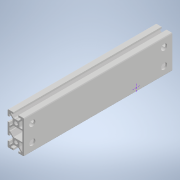
# Autodesk Inventor part: HFSF5-2040-180-LWH-RWH
Saved by Autodesk Inventor 2022 (Build 260153000, 153)
## iProperties
Category: PARTsolutions
Company: MISUMI
Created: 2022-12-05
Part Number: HFSF5-2040-180-LWH-RWH
Material: Generic
Catalog Web Link: www.cadenas.de
Description: NFS5-2040, NFSB5-2040, HFS5-2040, HFSB5-2040, CAF5-2040, NFSF5-2040, HFSF5-2040, HFSY5-2040-Aluminum Frames -5 Series-2Row Groove 20x40 mm Square -Specified Length
Vendor: MISUMI
Document SubType Name: Modeling
Designer: psAdmin
Manufacturer: MISUMI
Mass: 59.334 g
Surface Area: 583.137 cm^2
Volume: 59.334 cm^3
Density: 1 g/cm^3
Appearance: PSOLRGB-175-175-175
PSOL_IDENT_0: {$CADENAS_DATA/23d-libs/misumi/metric/38_al_extrusions_blackets/5/hfs5_2040.prj},644 {VTYP=3D},{NB=H
PSOL_IDENT_1: FSF5-2040-180-LWH-RWH},{LINA=HFSF5-2040-180-LWH-RWH},{NN=NFS5-2040, NFSB5-2040, HFS5-2040, HFSB5-204
PSOL_IDENT_2: 0, CAF5-2040, NFSF5-2040, HFSF5-2040, HFSY5-2040},{DATE=30.11.2021 06:05:55},{GEOMDATE=23.09.2021 02
PSOL_IDENT_3: :57:03},{VERSION=},{LINEID=30},{WBVAR=L,ALT1,ALT2,ALT4,ALT5,CP5,DL5,DR5,ALT6,ALT9,ALT10,ALT11,HP6,NH
PSOL_IDENT_4: L6,DL6,NHR6,DR6,ALT7,ALT8,NH9,AH,BH,CH,DH,EH,NH10,AV,BV,CV,DV,EV,NH11,AP,BP,CP,DP,EP,ALT12,ALT13,Z,N
PSOL_IDENT_5: H12,XA,XB,XC,XD,XE,NH13,YA,YB,YC,YD,YE,ALT16,HP16,DL16,DR16,ALT17,HQ17,JLP,ALT18,HQ18,KLP,ALT20},{WB
PSOL_IDENT_6: NUMERIC=L,NH9,AH,BH,CH,DH,EH,NH10,AV,BV,CV,DV,EV,NH11,AP,BP,CP,DP,EP,NH12,XA,XB,XC,XD,XE,NH13,YA,YB,
PSOL_IDENT_7: YC,YD,YE,HQ17,JLP,HQ18,KLP}  {NB=HFSF5-2040-180-LWH-RWH},{LINA=HFSF5-2040-180-LWH-RWH},{KT=DUMMY},{P
PSOL_IDENT_8: N=HFSF5-2040-180-LWH-RWH},{TPS=HFSF5-2040},{MAT=A6N01SS-T5 Aluminum Alloy},{ST=Clear Anodize},{FRMW=
PSOL_IDENT_9: 20},{FRMH=40},{FRD=4.2},{L=180},{MASS=0.93},{SA=344},{LX=1.52x10^4},{LY=5.40x10^4},{ALT1=},{M1=0},{D
PSOL_IDENT_10: PL1=0},{DPR1=0},{ALT1PN=},{ALT2=},{ALT2ALG= '','w/o End Tapping (Insert)','LHP','with LHP (Tapping o
PSOL_IDENT_11: n the Left (Insert))','RHP','with RHP (Tapping on the Right (Insert))','HPW','with HPW (Tapping on B
PSOL_IDENT_12: oth Ends (Insert))' },{M2=0},{DP2=0},{ALT2PN=},{ALT4=},{ALT4ALG= '', 'w/o SC (High Precision Cut)', '
PSOL_IDENT_13: SC', 'with SC (High Precision Cut)' },{ALT4PN=},{ALT5=},{ALT5ALG= '','w/o 45 Degree Cut','1','with 4
PSOL_IDENT_14: 5 Degree Cut' },{CP5=},{CP5ALG= '','N/A' },{DL5=},{DL5ALG= '','N/A' },{DR5=},{DR5ALG= '','N/A' },{FR
PSOL_IDENT_15: MLALT5=0},{FRMRALT5=0},{ALT5PN=},{ALT6=1},{ALT6ALG= '','w/o Fastening Location Wrench Access Hole Al
PSOL_IDENT_16: terations','1','with Fastening Location Wrench Access Hole Alterations' },{ALT9=},{ALT9ALG= '','w/o
PSOL_IDENT_17: Location Specified Wrench Access Hole Alteratons (Horizontal)','1','with Location Specified Wrench A
PSOL_IDENT_18: ccess Hole Alteratons (Horizontal)' },{ALT10=},{ALT10ALG= '','w/o Location Specified Wrench Access H
PSOL_IDENT_19: ole Alteratons (Vertical)','1','with Location Specified Wrench Access Hole Alteratons (Vertical)' },
PSOL_IDENT_20: {ALT11=},{ALT11ALG= '','w/o Location Specified Wrench Access Hole Alteratons (Crisscross)','1','with
PSOL_IDENT_21: Location Specified Wrench Access Hole Alteratons (Crisscross)' },{HP6=LR},{HP6ALG= 'L','Left','R','
PSOL_IDENT_22: Right','LR','Both Sides' },{NHL6=W},{NHL6ALG= 'C','C (Wrench Holes in Single Line)','W','W (Wrench H
PSOL_IDENT_23: oles in Two Lines)','E','E (Wrench Holes in Three Lines)' },{DL6=H},{DL6ALG= 'H','H (Horizontal)','V'
PSOL_IDENT_24: ,'V (Vertical)','P','P (Crisscross)' },{NHR6=W},{NHR6ALG= 'C','C (Wrench Holes in Single Line)','W','
PSOL_IDENT_25: W (Wrench Holes in Two Lines)','E','E (Wrench Holes in Three Lines)' },{DR6=H},{DR6ALG= 'H','H (Hori
PSOL_IDENT_26: zontal)','V','V (Vertical)','P','P (Crisscross)' },{HL6=10},{HL6D=10},{HR6=10},{HR6D=10},{J6=20},{J6
PSOL_IDENT_27: D=20},{K6=20},{K6D=0},{DD6=7.35},{DD6ALG=7.35},{ALT7=},{ALT7ALG= '','w/o FL (Shifts The Wrench Hole
PSOL_IDENT_28: on The Left Side 3mm Toward The Left End)','FL','with FL (Shifts The Wrench Hole on The Left Side 3m
PSOL_IDENT_29: m Toward The Left End)' },{ALT8=},{ALT8ALG= '','w/o FR (Shifts The Wrench Hole on The Right Side 3mm
PSOL_IDENT_30: Toward The Right End)','FR','with FR (Shifts The Wrench Hole on The Right Side 3mm Toward The Right
PSOL_IDENT_31: End)' },{ALT678PN=-LWH-RWH},{NH9=0},{NH9MAX=5},{NH9ALG=[0]},{AH=0.0},{AHMIN=7},{AHMAX=182.5},{AHALG=
PSOL_IDENT_32: [0]},{BH=0.0},{BHMIN=9.5},{BHMAX=192},{BHALG=[0]},{CH=0.0},{CHMIN=9.5},{CHMAX=201.5},{CHALG=[0]},{DH=
PSOL_IDENT_33: 0.0},{DHMIN=9.5},{DHMAX=211},{DHALG=[0]},{EH=0.0},{EHMIN=9.5},{EHMAX=173},{EHALG=[0]},{NH10=0},{NH10
PSOL_IDENT_34: MAX=5},{NH10ALG=[0]},{AV=0.0},{AVMIN=7},{AVMAX=182.5},{AVALG=[0]},{BV=0.0},{BVMIN=9.5},{BVMAX=192},{
PSOL_IDENT_35: BVALG=[0]},{CV=0.0},{CVMIN=9.5},{CVMAX=201.5},{CVALG=[0]},{DV=0.0},{DVMIN=9.5},{DVMAX=211},{DVALG=[0
PSOL_IDENT_36: ]},{EV=0.0},{EVMIN=9.5},{EVMAX=173},{EVALG=[0]},{NH11=0},{NH11MAX=5},{NH11ALG=[0]},{AP=0.0},{APMIN=7
PSOL_IDENT_37: },{APMAX=182.5},{APALG=[0]},{BP=0.0},{BPMIN=9.5},{BPMAX=192},{BPALG=[0]},{CP=0.0},{CPMIN=9.5},{CPMAX=
PSOL_IDENT_38: 201.5},{CPALG=[0]},{DP=0.0},{DPMIN=9.5},{DPMAX=211},{DPALG=[0]},{EP=0.0},{EPMIN=9.5},{EPMAX=173},{EP
PSOL_IDENT_39: ALG=[0]},{ALT9PN=},{ALT10PN=},{ALT11PN=},{ALT91011PN=},{ALT12=},{ALT12ALG= '','w/o Counterbore Hole
PSOL_IDENT_40: in Specified Position (Vertical)','1','with Counterbore Hole in Specified Position (Vertical)' },{AL
PSOL_IDENT_41: T13=},{ALT13ALG= '','N/A' },{Z=},{ZALG= '','N/A' },{DD12=0.0},{DD112=0.0},{NH12=0},{NH12MAX=5},{NH12
PSOL_IDENT_42: ALG=[0]},{XA=0.0},{XAMIN=7},{XAMAX=175},{XAALG=[0]},{XB=0.0},{XBMIN=2},{XBMAX=177},{XBALG=[0]},{XC=0
PSOL_IDENT_43: .0},{XCMIN=2},{XCMAX=179},{XCALG=[0]},{XD=0.0},{XDMIN=2},{XDMAX=181},{XDALG=[0]},{XE=0.0},{XEMIN=2},
PSOL_IDENT_44: {XEMAX=173},{XEALG=[0]},{NH13=0},{NH13MAX=5},{NH13ALG=[0]},{YA=0.0},{YAMIN=7},{YAMAX=175},{YAALG=[0]
PSOL_IDENT_45: },{YB=0.0},{YBMIN=2},{YBMAX=177},{YBALG=[0]},{YC=0.0},{YCMIN=2},{YCMAX=179},{YCALG=[0]},{YD=0.0},{YD
PSOL_IDENT_46: MIN=2},{YDMAX=181},{YDALG=[0]},{YE=0.0},{YEMIN=2},{YEMAX=173},{YEALG=[0]},{ALT12PN=},{ALT13PN=},{ALT
PSOL_IDENT_47: 1213PN=},{ALT16=},{ALT16ALG= '','w/o M Type Hole Alteration','1','with M Type Hole Alteration' },{HP
PSOL_IDENT_48: 16=},{HP16ALG= '','N/A' },{DL16=},{DL16ALG= '','N/A' },{DR16=},{DR16ALG= '','N/A' },{H116=0},{D16=0.
PSOL_IDENT_49: 0},{ALT16PN=},{ALT17=},{ALT17ALG= '','w/o L Type Hole Alteration (Top)','1','with L Type Hole Altera
PSOL_IDENT_50: tion (Top)' },{HQ17=0},{HQ17ALG=0},{JLP=0},{JLPMIN=4.9},{JLPMAX=0},{JLPALG=[0]},{L17=0},{D17=0.0},{A
PSOL_IDENT_51: LT18=},{ALT18ALG= '','w/o L Type Hole Alteration (Bottom)','1','with L Type Hole Alteration (Bottom)'
PSOL_IDENT_52: },{HQ18=0},{HQ18ALG=0},{KLP=0},{KLPMIN=4.9},{KLPMAX=0},{KLPALG=[0]},{L18=0},{D18=0.0},{ALT1718PN=},
PSOL_IDENT_53: {ALT20=},{ALT20PN=},{ERRORALT01=OK},{ERRORALT02=OK},{ERRORALT05=OK},{ERRORALT06091=OK},{ERRORALT0609
PSOL_IDENT_54: 2=OK},{ERRORALT06093=OK},{ERRORALT06094=OK},{ERRORALT06101=OK},{ERRORALT06102=OK},{ERRORALT06103=OK}
PSOL_IDENT_55: ,{ERRORALT06104=OK},{ERRORALT06111=OK},{ERRORALT06112=OK},{ERRORALT06113=OK},{ERRORALT06114=OK},{ERR
PSOL_IDENT_56: ORALT06121=OK},{ERRORALT06122=OK},{ERRORALT06123=OK},{ERRORALT06124=OK},{ERRORALT06131=OK},{ERRORALT
PSOL_IDENT_57: 06132=OK},{ERRORALT06133=OK},{ERRORALT06134=OK},{ERRORALT0616=OK},{ERRORALT06171=OK},{ERRORALT06172=
PSOL_IDENT_58: OK},{ERRORALT06173=OK},{ERRORALT06181=OK},{ERRORALT06182=OK},{ERRORALT06183=OK},{ERRORALT0911=OK},{E
PSOL_IDENT_59: RRORALT0913=OK},{ERRORALT0916=OK},{ERRORALT0917=OK},{ERRORALT0918=OK},{ERRORALT1011=OK},{ERRORALT101
PSOL_IDENT_60: 2=OK},{ERRORALT1016=OK},{ERRORALT1017=OK},{ERRORALT1018=OK},{ERRORALT1112=OK},{ERRORALT1113=OK},{ERR
PSOL_IDENT_61: ORALT1116=OK},{ERRORALT1117=OK},{ERRORALT1118=OK},{ERRORALT1216=OK},{ERRORALT1217=OK},{ERRORALT1218=
PSOL_IDENT_62: OK},{ERRORALT1316=OK},{ERRORALT1317=OK},{ERRORALT1318=OK},{ERRORALT1617=OK},{ERRORALT1618=OK},{ERROR
PSOL_IDENT_63: PN=},{TFW=2},{COLOR=}
NB: HFSF5-2040-180-LWH-RWH
NN: NFS5-2040, NFSB5-2040, HFS5-2040, HFSB5-2040, CAF5-2040, NFSF5-2040, HFSF5-2040, HFSY5-2040
NT: Aluminum Frames -5 Series-2Row Groove 20x40 mm Square -Specified Length
NBSYN: $PN.
LINA: HFSF5-2040-180-LWH-RWH
CATALOG: Misumi
PN: HFSF5-2040-180-LWH-RWH
TPS: HFSF5-2040
MAT: A6N01SS-T5 Aluminum Alloy
ST: Clear Anodize
L: 180
MASS: 0.93
SA: 344
LX: 1.52x10^4
LY: 5.40x10^4
ALT1: w/o End Tapping
M1: 0
DPL1: 0
DPR1: 0
ALT2: w/o End Tapping (Insert)
M2: 0
DP2: 0
ALT4: w/o SC (High Precision Cut)
ALT5: w/o 45 Degree Cut
CP5: N/A
DL5: N/A
DR5: N/A
ALT6: with Fastening Location Wrench Access Hole Alterations
ALT9: w/o Location Specified Wrench Access Hole Alteratons (Horizontal)
ALT10: w/o Location Specified Wrench Access Hole Alteratons (Vertical)
ALT11: w/o Location Specified Wrench Access Hole Alteratons (Crisscross)
HP6: Both Sides
NHL6: W (Wrench Holes in Two Lines)
DL6: H (Horizontal)
NHR6: W (Wrench Holes in Two Lines)
DR6: H (Horizontal)
HL6D: 10
HR6D: 10
J6D: 20
K6D: 0
DD6: 7.35
ALT7: w/o FL (Shifts The Wrench Hole on The Left Side 3mm Toward The Left End)
ALT8: w/o FR (Shifts The Wrench Hole on The Right Side 3mm Toward The Right End)
NH9: 0
AH: 0
BH: 0
CH: 0
DH: 0
EH: 0
NH10: 0
AV: 0
BV: 0
CV: 0
DV: 0
EV: 0
NH11: 0
AP: 0
BP: 0
CP: 0
DP: 0
EP: 0
ALT12: w/o Counterbore Hole in Specified Position (Vertical)
ALT13: N/A
Z: N/A
DD12: 0
DD112: 0
NH12: 0
XA: 0
XB: 0
XC: 0
XD: 0
XE: 0
NH13: 0
YA: 0
YB: 0
YC: 0
YD: 0
YE: 0
ALT16: w/o M Type Hole Alteration
HP16: N/A
DL16: N/A
DR16: N/A
H116: 0
D16: 0
ALT17: w/o L Type Hole Alteration (Top)
HQ17: 0
JLP: 0
D17: 0
ALT18: w/o L Type Hole Alteration (Bottom)
HQ18: 0
KLP: 0
D18: 0
ALT20: w/o CW (End Face C Chamfering)
SUPPLIER: MISUMI
ARTICLENO: HFSF5-2040-180-LWH-RWH
BOMINFO: HFSF5-2040-180-LWH-RWH
CREATOR: CADENAS GmbH
Title: HFSF5-2040-180-LWH-RWH
Author: Cadenas PARTsolutions
Comments: Aluminum Frames -5 Series-2Row Groove 20x40 mm Square -Specified Length
Autodesk Inventor part; units mm, degrees
sketch "Sketch_63" plane through (0, 0, 0) normal (0, 0, 1) x (1, 0, 0)
  line L0 (-10, -7) -> (-8, -7)
  line L1 (-8, -7) -> (-8, -4)
  line L2 (-8, -4) -> (-7.0607, -4)
  line L3 (-7.0607, -4) -> (-4, -7.0607)
  line L4 (-4, -7.0607) -> (-4, -9.4804)
  line L5 (-4, -9.4804) -> (-3.7, -10)
  line L6 (-3.7, -10) -> (-4, -10.5196)
  line L7 (-4, -10.5196) -> (-4, -12.9393)
  line L8 (-4, -12.9393) -> (-7.0607, -16)
  line L9 (-7.0607, -16) -> (-8, -16)
  line L10 (-8, -16) -> (-8, -13)
  line L11 (-8, -13) -> (-10, -13)
  line L12 (-10, -13) -> (-10, -19)
  arc A0 (-10, -19) -> (-9, -20) centre (-9, -19) ccw
  line L13 (-9, -20) -> (-3, -20)
  line L14 (-3, -20) -> (-3, -18)
  line L15 (-3, -18) -> (-6, -18)
  line L16 (-6, -18) -> (-6, -17.0607)
  line L17 (-6, -17.0607) -> (-2.9393, -14)
  line L18 (-2.9393, -14) -> (-0.5196, -14)
  line L19 (-0.5196, -14) -> (0, -13.7)
  line L20 (0, -13.7) -> (0.5196, -14)
  line L21 (0.5196, -14) -> (2.9393, -14)
  line L22 (2.9393, -14) -> (6, -17.0607)
  line L23 (6, -17.0607) -> (6, -18)
  line L24 (6, -18) -> (3, -18)
  line L25 (3, -18) -> (3, -20)
  line L26 (3, -20) -> (9, -20)
  arc A1 (9, -20) -> (10, -19) centre (9, -19) ccw
  line L27 (10, -19) -> (10, 19)
  arc A2 (10, 19) -> (9, 20) centre (9, 19) ccw
  line L28 (9, 20) -> (3, 20)
  line L29 (3, 20) -> (3, 18)
  line L30 (3, 18) -> (6, 18)
  line L31 (6, 18) -> (6, 17.0607)
  line L32 (6, 17.0607) -> (2.9393, 14)
  line L33 (2.9393, 14) -> (0.5196, 14)
  line L34 (0.5196, 14) -> (0, 13.7)
  line L35 (0, 13.7) -> (-0.5196, 14)
  line L36 (-0.5196, 14) -> (-2.9393, 14)
  line L37 (-2.9393, 14) -> (-6, 17.0607)
  line L38 (-6, 17.0607) -> (-6, 18)
  line L39 (-6, 18) -> (-3, 18)
  line L40 (-3, 18) -> (-3, 20)
  line L41 (-3, 20) -> (-9, 20)
  arc A3 (-9, 20) -> (-10, 19) centre (-9, 19) ccw
  line L42 (-10, 19) -> (-10, 13)
  line L43 (-10, 13) -> (-8, 13)
  line L44 (-8, 13) -> (-8, 16)
  line L45 (-8, 16) -> (-7.0607, 16)
  line L46 (-7.0607, 16) -> (-4, 12.9393)
  line L47 (-4, 12.9393) -> (-4, 10.5196)
  line L48 (-4, 10.5196) -> (-3.7, 10)
  line L49 (-3.7, 10) -> (-4, 9.4804)
  line L50 (-4, 9.4804) -> (-4, 7.0607)
  line L51 (-4, 7.0607) -> (-7.0607, 4)
  line L52 (-7.0607, 4) -> (-8, 4)
  line L53 (-8, 4) -> (-8, 7)
  line L54 (-8, 7) -> (-10, 7)
  line L55 (-10, 7) -> (-10, -7)
  line L56 (4, 12.9393) -> (4, 8.5)
  arc A4 (4, 8.5) -> (5, 7.5) centre (5, 8.5) ccw
  line L57 (5, 7.5) -> (7, 7.5)
  arc A5 (7, 7.5) -> (8, 8.5) centre (7, 8.5) ccw
  line L58 (8, 8.5) -> (8, 16)
  line L59 (8, 16) -> (7.0607, 16)
  line L60 (7.0607, 16) -> (4, 12.9393)
  line L61 (4, -12.9393) -> (7.0607, -16)
  line L62 (7.0607, -16) -> (8, -16)
  line L63 (8, -16) -> (8, -8.5)
  arc A6 (8, -8.5) -> (7, -7.5) centre (7, -8.5) ccw
  line L64 (7, -7.5) -> (5, -7.5)
  arc A7 (5, -7.5) -> (4, -8.5) centre (5, -8.5) ccw
  line L65 (4, -8.5) -> (4, -12.9393)
  line L66 (-8, 1.7) -> (-8, -1.7)
  arc A8 (-8, -1.7) -> (-7.7, -2) centre (-7.7, -1.7) ccw
  line L67 (-7.7, -2) -> (-7.0636, -2)
  arc A9 (-6.8515, -2.0879) -> (-7.0636, -2) centre (-7.0636, -2.3) ccw
  line L68 (-6.8515, -2.0879) -> (-2.9393, -6)
  line L69 (-2.9393, -6) -> (7, -6)
  arc A10 (7, -6) -> (8, -5) centre (7, -5) ccw
  line L70 (8, -5) -> (8, 5)
  arc A11 (8, 5) -> (7, 6) centre (7, 5) ccw
  line L71 (7, 6) -> (-2.9393, 6)
  line L72 (-2.9393, 6) -> (-6.8515, 2.0879)
  arc A12 (-7.0636, 2) -> (-6.8515, 2.0879) centre (-7.0636, 2.3) ccw
  line L73 (-7.0636, 2) -> (-7.7, 2)
  arc A13 (-7.7, 2) -> (-8, 1.7) centre (-7.7, 1.7) ccw
  constraints: 148 end point, 28 point on circle, 14 centre point
extrude "Extrusion1" add sketch "Sketch_63" against normal blind 180
sketch "Sketch2" plane through (0, 0, -180) normal (0, 0, -1) x (-1, 0, 0)
  point P0 (0, 10)
hole "Hole1" at (0, 10, -180) direction (0, 0, 1) diameter 4.2 depth 180
pattern_linear "Rectangular Pattern1" count 2 spacing 20 along (0, -1, 0) of "Hole1"
sketch "Sketch3" plane through (10, -19, 0) normal (1, 0, 0) x (0, 0, -1)
  point P0 (10, 29)
hole "Hole2" at (10, 10, -10) direction (-1, 0, 0) diameter 7.35 depth 20
sketch "Sketch4" plane through (10, -19, 0) normal (1, 0, 0) x (0, 0, -1)
  point P0 (10, 9)
hole "Hole3" at (10, -10, -10) direction (-1, 0, 0) diameter 7.35 depth 20
sketch "Sketch7" plane through (10, -19, 0) normal (1, 0, 0) x (0, 0, -1)
  point P0 (170, 29)
hole "Hole6" at (10, 10, -170) direction (-1, 0, 0) diameter 7.35 depth 20
sketch "Sketch8" plane through (10, -19, 0) normal (1, 0, 0) x (0, 0, -1)
  point P0 (170, 9)
hole "Hole7" at (10, -10, -170) direction (-1, 0, 0) diameter 7.35 depth 20
ref_plane "C1_XY" through (0, 0, 0) normal (0, 0, 1) x (1, 0, 0)
ref_plane "C1_YZ" through (0, 0, 0) normal (1, 0, 0) x (0, 1, 0)
ref_plane "C1_ZX" through (0, 0, 0) normal (0, 1, 0) x (0, 0, 1)
sketch "スケッチ10" plane through (10, -19, 0) normal (1, 0, 0) x (0, 0, -1)
  line L0 (0, 0) -> (180, 0) projected
  line L1 (0, 0) -> (0, 38) projected
  point P0 (136, 3)
  point P1 (116, 3)
  point P2 (136, 27)
  point P3 (116, 27)
  dimension "d65" = 3
  dimension "d66" = 136
  dimension "d69" = 20
  dimension "d72" = 24
  constraints: 1 horizontal, 1 vertical, 3 other
  measures "d65" distance from line of point (136, 3) L0
  measures "d66" distance from line of L1 point (136, 3)
  measures "d69" distance of point (136, 3) point (116, 3)
  measures "d72" distance of point (136, 3) point (136, 27)
hole "穴9" at (10, -16, -136) at (10, -16, -116) at (10, 8, -136) at (10, 8, -116) direction (-1, 0, 0) diameter 3.2 end through all
body "Solid1"
